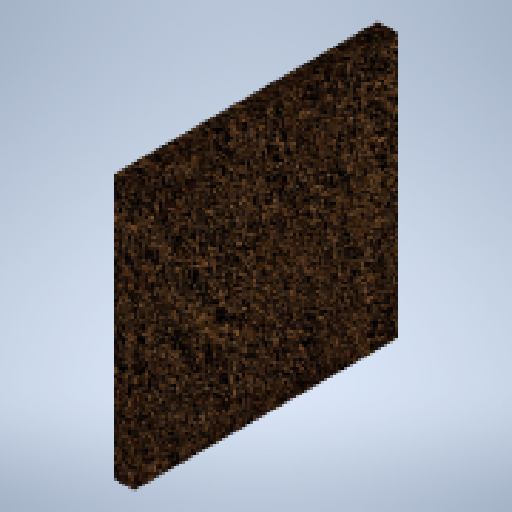
# Autodesk Inventor part: base horiz
Saved by Autodesk Inventor 2023 (Build 270158000, 158)
## iProperties
Created: 2023-03-27
Part Number: base horiz
Material: Generic
Document SubType Name: Modeling
Designer: sebas
Density: 1 g/cm^3
Appearance: Dirt - Dark Brown
Author: sebas
Autodesk Inventor part; units mm, degrees
ref_plane "YZ Plane" through (0, 0, 0) normal (1, 0, 0) x (0, 1, 0)
ref_plane "XZ Plane" through (0, 0, 0) normal (0, 1, 0) x (-1, 0, 0)
ref_plane "XY Plane" through (0, 0, 0) normal (0, 0, 1) x (1, 0, 0)
sketch "Sketch1" plane through (0, 0, 0) normal (0, 1, 0) x (-1, 0, 0)
  line L0 (0, 0) -> (19.05, 0)
  line L1 (19.05, 0) -> (19.05, -250)
  line L2 (19.05, -250) -> (0, -250)
  line L3 (0, -250) -> (0, 0)
  dimension "d0" = 19.05
  dimension "d1" = 250
  constraints: 8 end point, 3 perpendicular, 1 horizontal
  measures "d0" distance of L0.start L0.end
  measures "d1" distance of L0.end L1.end
extrude "Extrusion1" add sketch "Sketch1" along normal blind 250
body "Solid1"
